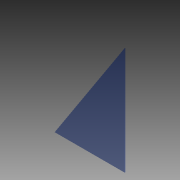
# Autodesk Inventor part: side window
Saved by Autodesk Inventor 2012 (Build 160160000, 160)
## iProperties
Created: 2011-12-02
Part Number: side window
Material: Polycarbonate, Clear
Document SubType Name: Modeling
Designer: Antonella
Mass: 31.7711 g
Surface Area: 343.682 cm^2
Volume: 26.4759 cm^3
Density: 1.2 g/cm^3
Author: Antonella
Autodesk Inventor part; units mm, degrees
ref_plane "YZ Plane" through (0, 0, 0) normal (1, 0, 0) x (0, 1, 0)
ref_plane "XZ Plane" through (0, 0, 0) normal (0, 1, 0) x (-1, 0, 0)
ref_plane "XY Plane" through (0, 0, 0) normal (0, 0, 1) x (1, 0, 0)
sketch "Sketch1" plane through (0, 0, 0) normal (0, 0, 1) x (1, 0, 0)
  line L0 (-198.12, 0) -> (33.02, 0) projected
  line L1 (0, -50.8463) -> (0, 305.078) projected
  line L2 (0, 254.2317) -> (0, 0)
  line L3 (0, 0) -> (-165.1, 0)
  line L4 (-165.1, 0) -> (0, 254.2317)
  point P0 (0, 0)
  dimension "d0" = 165.1
  dimension "d4" = 57
  constraints: 6 end point, 3 collinear, 1 perpendicular
  measures "d0" distance of L2.end L3.end
  measures "d4" angle of L4 L0
extrude "Extrusion1" add sketch "Sketch1" along normal blind 1.5875
body "Solid1"
